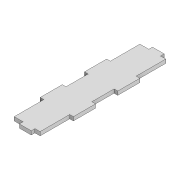
# Autodesk Inventor part: Lat 1
Saved by Autodesk Inventor 2022 (Build 260153000, 153)
## iProperties
Created: 2022-06-21
Part Number: Lat 1
Material: Generic
Document SubType Name: Modeling
Designer: ADMIN
Density: 1 g/cm^3
Appearance: Default
Author: ADMIN
Autodesk Inventor part; units mm, degrees
ref_plane "YZ Plane" through (0, 0, 0) normal (1, 0, 0) x (0, 1, 0)
ref_plane "XZ Plane" through (0, 0, 0) normal (0, 1, 0) x (-1, 0, 0)
ref_plane "XY Plane" through (0, 0, 0) normal (0, 0, 1) x (1, 0, 0)
sketch "Sketch1" plane through (0, 0, 0) normal (0, 1, 0) x (-1, 0, 0)
  line L0 (-89.6269, -268.05) -> (-54.6269, -268.05)
  line L1 (-54.6269, -268.05) -> (-54.6269, -98.05)
  line L2 (-54.6269, -98.05) -> (-89.6269, -98.05)
  line L3 (-89.6269, -98.05) -> (-89.6269, -268.05)
  line L4 (-82.6269, -268.05) -> (-66.6269, -268.05)
  line L5 (-66.6269, -268.05) -> (-66.6269, -273.05)
  line L6 (-66.6269, -273.05) -> (-82.6269, -273.05)
  line L7 (-82.6269, -273.05) -> (-82.6269, -268.05)
  line L8 (-89.6269, -228.05) -> (-94.6269, -228.05)
  line L9 (-94.6269, -228.05) -> (-94.6269, -198.05)
  line L10 (-94.6269, -198.05) -> (-89.6269, -198.05)
  line L11 (-89.6269, -198.05) -> (-89.6269, -228.05)
  line L12 (-89.6269, -168.05) -> (-94.6269, -168.05)
  line L13 (-94.6269, -168.05) -> (-94.6269, -138.05)
  line L14 (-94.6269, -138.05) -> (-89.6269, -138.05)
  line L15 (-89.6269, -138.05) -> (-89.6269, -168.05)
  line L16 (-72.1269, -98.05) -> (-72.1269, -268.05)
  line L17 (-54.6269, -228.05) -> (-49.6269, -228.05)
  line L18 (-49.6269, -228.05) -> (-49.6269, -198.05)
  line L19 (-49.6269, -198.05) -> (-54.6269, -198.05)
  line L20 (-54.6269, -198.05) -> (-54.6269, -228.05)
  line L21 (-54.6269, -168.05) -> (-49.6269, -168.05)
  line L22 (-49.6269, -168.05) -> (-49.6269, -138.05)
  line L23 (-49.6269, -138.05) -> (-54.6269, -138.05)
  line L24 (-54.6269, -138.05) -> (-54.6269, -168.05)
  line L25 (-82.6269, -98.05) -> (-66.6269, -98.05)
  line L26 (-66.6269, -98.05) -> (-66.6269, -93.05)
  line L27 (-66.6269, -93.05) -> (-82.6269, -93.05)
  line L28 (-82.6269, -93.05) -> (-82.6269, -98.05)
  dimension "d22" = 35
  dimension "d23" = 170
  dimension "d24" = 16
  dimension "d25" = 5
  dimension "d26" = 12
  dimension "d27" = 5
  dimension "d28" = 30
  dimension "d29" = 5
  dimension "d30" = 30
  dimension "d31" = 30
  dimension "d32" = 40
  dimension "d33" = 5
  dimension "d34" = 16
  dimension "d35" = 5
  constraints: 58 end point, 14 parallel, 8 perpendicular, 8 point on line, 7 horizontal, 1 midpoint
  measures "d22" distance of L2.end L1.end
  measures "d23" distance of L1.end L0.end
  measures "d24" distance of L5.end L6.end
  measures "d25" distance of L4.end L5.end
  measures "d26" distance between parallel lines of L1 L5
  measures "d27" distance of L9.end L10.end
  measures "d28" distance of L8.end L9.end
  measures "d29" distance of L13.end L14.end
  measures "d30" distance of L12.end L13.end
  measures "d31" distance between parallel lines of L12 L10
  measures "d32" distance between parallel lines of L0 L8
  measures "d33" distance of L19.end L18.end
  measures "d34" distance of L27.end L26.end
  measures "d35" distance of L26.end L25.end
extrude "Extrusion2" add sketch "Sketch1" along normal blind 5
body "Solid2"
